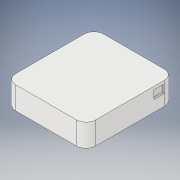
# Autodesk Inventor part: Yoobao
Saved by Autodesk Inventor 2019 (Build 230136000, 136)
## iProperties
Created: 2019-02-12
Part Number: Yoobao
Material: Generic
Document SubType Name: Modeling
Designer: izsoandras
Density: 1 g/cm^3
Appearance: Default
Author: izsoandras
Autodesk Inventor part; units mm, degrees
ref_plane "YZ Plane" through (0, 0, 0) normal (1, 0, 0) x (0, 1, 0)
ref_plane "XZ Plane" through (0, 0, 0) normal (0, 1, 0) x (-1, 0, 0)
ref_plane "XY Plane" through (0, 0, 0) normal (0, 0, 1) x (1, 0, 0)
sketch "Sketch1" plane through (0, 0, 0) normal (0, 1, 0) x (-1, 0, 0)
  line L0 (22.5526, 63.1659) -> (-40.8374, 63.1659)
  line L1 (-50.8374, 53.1659) -> (-50.8374, -18.3141)
  line L2 (-40.8374, -28.3141) -> (22.5526, -28.3141)
  line L3 (32.5526, -18.3141) -> (32.5526, 53.1659)
  arc A0 (32.5526, 53.1659) -> (22.5526, 63.1659) centre (22.5526, 53.1659) ccw
  arc A1 (22.5526, -28.3141) -> (32.5526, -18.3141) centre (22.5526, -18.3141) ccw
  arc A2 (-50.8374, -18.3141) -> (-40.8374, -28.3141) centre (-40.8374, -18.3141) ccw
  arc A3 (-40.8374, 63.1659) -> (-50.8374, 53.1659) centre (-40.8374, 53.1659) ccw
  point P0 (0, 0)
  point P1 (32.5526, 63.1659)
  point P2 (-50.8374, 63.1659)
  point P3 (32.5526, -28.3141)
  dimension "d0" = 83.39
  dimension "d1" = 91.48
  dimension "d2" = 10
  dimension "d3" = 10
  constraints: 8 end point, 8 point on circle, 8 tangent, 6 point on line, 4 centre point, 2 equal radius, 2 parallel, 1 horizontal, 1 perpendicular
  measures "d0" distance of point (32.553, 63.166) point (-50.837, 63.166)
  measures "d1" distance of point (32.553, -28.314) point (32.553, 63.166)
  measures "d2" radius of A0
  measures "d3" radius of A1
extrude "Extrusion1" add sketch "Sketch1" along normal blind 23.54
sketch "Sketch2" plane through (40.8374, 0, -28.3141) normal (0, 0, -1) x (-1, 0, 0)
  line L0 (7.595, 14.9788) -> (21.095, 14.9788)
  line L1 (21.095, 14.9788) -> (21.095, 8.3788)
  line L2 (21.095, 8.3788) -> (7.595, 8.3788)
  line L3 (7.595, 8.3788) -> (7.595, 14.9788)
  line L4 (42.295, 14.9788) -> (55.795, 14.9788)
  line L5 (55.795, 14.9788) -> (55.795, 8.3788)
  line L6 (55.795, 8.3788) -> (42.295, 8.3788)
  line L7 (42.295, 8.3788) -> (42.295, 14.9788)
  line L8 (73.39, 0) -> (73.39, 23.54) projected
  point P0 (40.8374, 0)
  dimension "d6" = 13.5
  dimension "d7" = 6.6
  dimension "d8" = 13.5
  dimension "d9" = 6.6
  dimension "d10" = 21.2
  dimension "d11" = 17.595
  constraints: 16 end point, 4 parallel, 2 horizontal, 2 perpendicular
  measures "d6" distance of L1.end L2.end
  measures "d7" distance of L2.end L0.start
  measures "d8" distance of L4.start L4.end
  measures "d9" distance of L6.end L4.start
  measures "d10" distance between parallel lines of L1 L7
  measures "d11" distance between parallel lines of L8 L5
extrude "Extrusion2" cut sketch "Sketch2" against normal blind 5
sketch "Sketch3" plane through (40.8374, 0, -28.3141) normal (0, 0, -1) x (-1, 0, 0)
  circle A0 centre (31.695, 11.77) radius 3
  line L0 (0, 23.54) -> (63.39, 23.54) projected
  line L1 (-10, 0) -> (-10, 23.54) projected
  point P0 (40.8374, 0)
  dimension "d14" = 6
  dimension "d15" = 11.77
  dimension "d16" = 41.695
  constraints: 1 centre point
  measures "d14" diameter of A0
  measures "d15" distance from line of L0 A0.centre
  measures "d16" distance from line of L1 A0.centre
extrude "Extrusion3" cut sketch "Sketch3" against normal blind 2
sketch "Sketch4" plane through (-32.5526, 0, -18.3141) normal (-1, 0, 0) x (0, 0, 1)
  line L0 (0, 15.77) -> (9.2, 15.77)
  line L1 (9.2, 15.77) -> (9.2, 11.77)
  line L2 (9.2, 11.77) -> (0, 11.77)
  line L3 (0, 11.77) -> (0, 15.77)
  line L4 (0, 0) -> (0, 23.54) projected
  line L5 (71.48, 0) -> (0, 0) projected
  point P0 (18.3141, 0)
  dimension "d19" = 9.2
  dimension "d20" = 4
  dimension "d21" = 0
  dimension "d22" = 11.77
  constraints: 8 end point, 2 parallel, 1 horizontal, 1 perpendicular
  measures "d19" distance of L1.end L2.end
  measures "d20" distance of L0.end L1.end
  measures "d21" distance between parallel lines of L4 L3
  measures "d22" distance between parallel lines of L5 L2
extrude "Extrusion4" cut sketch "Sketch4" against normal blind 3
sketch "Sketch5" plane through (50.8374, 0, 53.1659) normal (1, 0, 0) x (0, 0, -1)
  line L0 (71.48, 15.77) -> (71.48, 23.54) projected
  line L1 (71.48, 20.37) -> (60.68, 20.37)
  line L2 (60.68, 20.37) -> (60.68, 11.77)
  line L3 (60.68, 11.77) -> (71.48, 11.77)
  line L4 (71.48, 11.77) -> (71.48, 20.37)
  line L5 (71.48, 0) -> (0, 0) projected
  point P0 (53.1659, 0)
  dimension "d25" = 8.6
  dimension "d26" = 10.8
  dimension "d27" = 11.77
  constraints: 8 end point, 2 parallel, 1 horizontal, 1 perpendicular, 1 point on line
  measures "d25" distance of L1.end L2.end
  measures "d26" distance of L1.start L1.end
  measures "d27" distance between parallel lines of L5 L3
extrude "Extrusion5" cut sketch "Sketch5" against normal blind 2
equation "\"d8\" = d6"
equation "\"d9\" = d7"
equation "\"d11\" = -d6 + 0.5 * d0 - 0.5 * d10"
equation "\"d16\" = 0.5 * d0"
body "Solid1"
